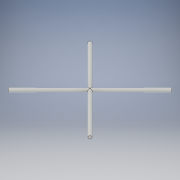
# Autodesk Inventor part: CrossbeamPoleAJB
Saved by Autodesk Inventor 2018 (Build 220112000, 112)
## iProperties
Created: 2018-02-16
Part Number: CrossbeamPoleAJB
Material: Generic
Document SubType Name: Modeling
Designer: Alec temporary
Density: 1 g/cm^3
Appearance: Default
Author: Alec temporary
Autodesk Inventor part; units mm, degrees
sketch "Sketch1" plane through (0, 0, 0) normal (0, 0, 1) x (1, 0, 0)
  line L0 (-1895.2334, -130.644) -> (-1895.2334, 123.356) projected
  line L1 (1914.7078, -105.244) -> (1914.7078, 97.956) projected
  line L2 (1609.9078, 123.356) -> (1609.9078, -130.644) projected
  line L3 (1609.9078, -3.644) -> (1762.3078, -3.644)
  line L4 (1914.7078, -3.644) -> (5115.049, -3.644) construction
  line L5 (5115.049, -130.644) -> (5115.049, 123.356) projected
  line L6 (1914.7078, -3.644) -> (3514.8784, -3.644) construction
  line L7 (1609.9078, -130.644) -> (5115.049, -130.644)
  line L8 (1609.9078, 130.644) -> (5115.049, 130.644)
  line L9 (0, 0) -> (3514.8784, 0) construction
  line L10 (3514.8784, 0) -> (3514.8784, 27.5413)
  dimension "d0" = 304.8
  dimension "d1" = 152.4
  dimension "d2" = 3200.3412
  dimension "d3" = 1600.1706
  dimension "d4" = 261.2879
  dimension "d5" = 3514.8784
  constraints: 14 end point, 5 horizontal, 4 midpoint, 1 coincident, 1 vertical, 2 other
  measures "d0" distance between parallel lines of L1 L2
  measures "d1" distance of L3.start L3.end
  measures "d2" distance of L4.start L4.end
  measures "d3" distance of L4.start L6.end
  measures "d4" distance between parallel lines of L8 L7
  measures "d5" distance of L9.start L9.end
ref_plane "Work Plane1" through (3514.8784, 0, 0) normal (-0.7071, 0, 0.7071) x (0, 1, 0)
sketch "Sketch2" plane through (3514.8784, 0, 0) normal (-0.7071, 0, 0.7071) x (0, 1, 0)
  circle A0 centre (0, 0) radius 50.8
  point P0 (0, 2485.3943)
  dimension "d7" = 101.6
  constraints: 1 centre point, 1 coincident
  measures "d7" diameter of A0
extrude "Extrusion1" add sketch "Sketch2" against normal blind 3810
sketch "Sketch3" plane through (0, 0, 0) normal (0, 1, 0) x (-1, 0, 0)
  line L0 (-14897.9748, 11383.0964) -> (3194.7063, -6709.5846) construction
  line L1 (-18516.511, 0) -> (6813.2425, 0) construction
  line L2 (-820.8015, 0) -> (-2167.8399, -1347.0384) construction
  line L3 (-3550.7994, 35.921) -> (-3478.9573, -35.921) construction
  line L4 (-3514.8784, 0) -> (-820.8015, -2694.0768) construction
  point P0 (0, 0)
  dimension "d10" = 3810
  dimension "d11" = 1905
  constraints: 6 end point, 2 point on line, 1 collinear, 1 midpoint, 1 perpendicular, 3 other
  measures "d10" distance of L4.start L4.end
  measures "d11" distance of L2.start L2.end
sketch "Sketch4" plane through (0, 0, 0) normal (0, 0, 1) x (1, 0, 0)
  line L0 (820.8015, 0) -> (820.8015, 41.7807)
  point P0 (0, 0)
  constraints: 2 end point, 1 vertical
ref_plane "Work Plane2" through (820.8015, 0, 0) normal (0.7071, 0, 0.7071) x (0, 1, 0)
ref_plane "Work Plane6" through (4861.9168, 0, -1347.0384) normal (-0.7071, 0, 0.7071) x (0, 1, 0)
ref_plane "Work Plane7" through (820.8015, 0, -2694.0768) normal (0, 0, -1) x (0, 1, 0)
ref_plane "Work Plane8" through (3514.8784, 0, -2694.0768) normal (1, 0, 0) x (0, 1, 0)
sketch "Sketch5" plane through (820.8015, 0, 0) normal (0.7071, 0, 0.7071) x (0, 1, 0)
  line L0 (-182.9016, -3810) -> (182.9016, -3810) projected
  line L1 (0, 580.3943) -> (0, -3810)
  circle A0 centre (0, -3810) radius 50.8
  dimension "d17" = 101.6
  constraints: 2 coincident, 2 end point, 1 centre point, 1 midpoint, 1 vertical
  measures "d17" diameter of A0
extrude "Extrusion2" add sketch "Sketch5" along normal blind 3810
ref_plane "Work Plane3" through (820.8015, 0, 0) normal (1, 0, 0) x (0, 1, 0)
ref_plane "Work Plane4" through (-526.2369, 0, -1347.0384) normal (0.7071, 0, 0.7071) x (0, 1, 0)
ref_plane "Work Plane5" through (3514.8784, 0, 0) normal (-0.7071, 0, 0.7071) x (0, 1, 0)
equation "\"d3\" = 0.5 * d2"
body "Solid1"
